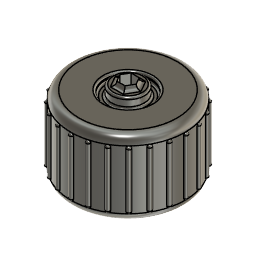
MEH01 Roller - mod (Autodesk Fusion 360 design; units mm, degrees)
Autodesk Fusion 360 part; units mm, degrees
sketch "Sketch1" plane through (0, 0, 0) normal (0, 0, 1) x (1, 0, 0)
  circle A0 centre (0, 0) radius 7
  circle A1 centre (0, 0) radius 3
  circle A2 centre (0.0729, -6.9996) radius 0.25
  dimension "d1" = 14
  dimension "d4" = 6
  dimension "d30" = 0.5
  constraint coincident A0.centre A1.centre
  constraint concentric A0 A1
  constraint coincident A0 A2.centre
  measures "d1" diameter of A0
  measures "d4" diameter of A1
  measures "d30" diameter of A2
extrude "Extrude1" add sketch "Sketch1" along normal blind 9.2 contours A0 A2 | A0 A2 | A1 picked at (-0.6353, -5.5331) picked at (0.0782, -6.9161) makes body 1
extrude "Extrude2" cut sketch "Sketch1" along normal blind 2 contours A1 bodies 1
sketch "Sketch2" plane through (0, 0, 0) normal (0, 0, 1) x (1, 0, 0)
  circle A0 centre (0, 0) radius 2
  dimension "d7" = 4
  constraint coincident A0.centre origin
  measures "d7" diameter of A0
extrude "Extrude3" cut sketch "Sketch2" along normal blind 2 from surface at 2 bodies 1
sketch "Sketch3" plane through (0, 0, 9.2) normal (0, 0, 1) x (-1, 0, 0)
  line L0 (-0.5023, 0.87) -> (-1.0046, 0)
  line L1 (-1.0046, 0) -> (-0.5023, -0.87)
  line L2 (-0.5023, -0.87) -> (0.5023, -0.87)
  line L3 (0.5023, -0.87) -> (1.0046, 0)
  line L4 (1.0046, 0) -> (0.5023, 0.87)
  line L5 (0.5023, 0.87) -> (-0.5023, 0.87)
  circle A0 centre (0, 0) radius 2.8
  circle A1 centre (0, 0) radius 2
  dimension "d11" = 0.87
  dimension "d16" = 5.6
  dimension "d19" = 4
  constraint coincident A0.centre A1.centre
  constraint concentric A0 A1
  measures "d11" distance of A0.centre L5
  measures "d16" diameter of A0
  measures "d19" diameter of A1
extrude "Extrude5" cut sketch "Sketch3" against normal blind 0.64 contours A0 | A1 bodies 1
extrude "Extrude6" add sketch "Sketch3" along normal blind 0.64 from surface at -0.64 contours A1 bodies 1
extrude "Extrude7" add sketch "Sketch3" along normal blind 0.6 contours A1 bodies 1
extrude "Extrude8" add sketch "Sketch3" along normal blind 2.4 contours L0 L1 L2 L3 L4 L5 bodies 1
fillet "Fillet2" radius 0.5 6 edges at (0, -0.87, 9.8) (-0.7534, -0.435, 9.8) (0.7534, -0.435, 9.8) (0.7534, 0.435, 9.8) (0, 0.87, 9.8) (-0.7534, 0.435, 9.8) on bodies 1
fillet "Fillet3" radius 1 2 edges at (-6.5263, -2.5313, 9.2) (-6.5263, -2.5313, 0) on bodies 1
extrude "Extrude9" add sketch "Sketch1" along normal blind 7.2 from surface at 1 separate body contours A0 A2 picked at (0.0788, -7.0824) makes body 2
fillet "Fillet4" radius 0.25 2 edges at (0.0755, -7.2496, 8.2) (0.0755, -7.2496, 1) on bodies 2
pattern_circular "C-Pattern1" count 24 over 360 about axis through (0, 0, 1.75) along (0, 0, 1) of bodies 2 makes body 3 at (2.1217, -6.8133, 5.7167) makes body 4 at (3.7854, -5.9114, 5.7167) makes body 5 at (4.9778, -5.1469, 5.7167) makes body 6 at (6.234, -3.2267, 5.7167) makes body 7 at (6.8567, -1.5033, 5.7167) makes body 8 at (7.0952, -0.1581, 5.7167) makes body 9 at (6.9134, 1.6998, 5.7167) makes body 10 at (5.9226, 3.7908, 5.7167) makes body 11 at (5.0709, 5.1815, 5.7167) makes body 12 at (3.2267, 6.234, 5.7167) makes body 13 at (1.5033, 6.8567, 5.7167) makes body 14 at (0.1581, 7.0952, 5.7167) makes body 15 at (-1.6998, 6.9134, 5.7167) makes body 16 at (-3.7854, 5.9114, 5.7167) makes body 17 at (-5.1946, 4.7397, 5.7167) makes body 18 at (-6.234, 3.2267, 5.7167) makes body 19 at (-6.8567, 1.5033, 5.7167) makes body 20 at (-7.0952, 0.1581, 5.7167) makes body 21 at (-6.9462, -1.7375, 5.7167) makes body 22 at (-5.9114, -3.7854, 5.7167) makes body 23 at (-5.1469, -4.9778, 5.7167) makes body 24 at (-3.2267, -6.234, 5.7167) makes body 25 at (-1.5033, -6.8567, 5.7167)
combine "Combine1" operation add target body 1 tool bodies 2 14 17 20 3 23 13 18 5 10 7 11 16 4 6 8 9 12 15 19 21 22 24 25
fillet "Fillet5" radius 0.24 1 edges at (1.8647, 0.7232, 9.8) on bodies 1
fillet "Fillet6" radius 0.24 2 edges at (2.6105, -1.0125, 8.56) (1.8647, -0.7232, 8.56) on bodies 1
fillet "Fillet7" radius 0.24 1 edges at (2.6105, -1.0125, 9.2) on bodies 1
extrude "Extrude10" cut 1 faces at (0.3349, 0, 11.6) along direction (0, 0, -1) blind 8 on bodies 1 bodies 1
equation "d11 = ( 1.74 / 2 ) * 1 mm"
